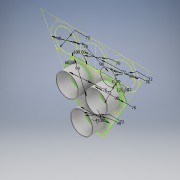
# Autodesk Inventor part: base
Saved by Autodesk Inventor 2019 (Build 230136000, 136)
## iProperties
Created: 2020-09-26
Part Number: base
Material: Generic
Document SubType Name: Modeling
Designer: Obscure_Decision
Density: 1 g/cm^3
Appearance: Default
Author: Obscure_Decision
Autodesk Inventor part; units mm, degrees
ref_plane "YZ Plane" through (0, 0, 0) normal (1, 0, 0) x (0, 1, 0)
ref_plane "XZ Plane" through (0, 0, 0) normal (0, 1, 0) x (-1, 0, 0)
ref_plane "XY Plane" through (0, 0, 0) normal (0, 0, 1) x (1, 0, 0)
sketch "Sketch1" plane through (0, 0, 0) normal (0, 0, 1) x (1, 0, 0)
  circle A0 centre (0, 0) radius 49 construction
  line L0 (0, 0) -> (49, 0) construction
  circle A1 centre (49, 84.8705) radius 49 construction
  circle A2 centre (-49, 84.8705) radius 49 construction
  circle A3 centre (0, 169.741) radius 49 construction
  circle A4 centre (-98, 169.741) radius 49 construction
  circle A5 centre (98, 169.741) radius 49 construction
  circle A6 centre (-49, 84.8705) radius 36
  circle A7 centre (-98, 169.741) radius 36 construction
  circle A8 centre (0, 169.741) radius 36 construction
  circle A9 centre (98, 169.741) radius 36 construction
  circle A10 centre (49, 84.8705) radius 36
  circle A11 centre (0, 0) radius 36
  line L1 (0, 0) -> (34.6482, -34.6482) construction
  line L2 (0, 0) -> (49, 0) construction
  line L3 (-183.7192, 220.2111) -> (183.7192, 220.2111) construction
  line L4 (-52.5602, 133.741) -> (45.4398, 133.741) construction
  line L5 (-52.5602, 133.741) -> (-77.2006, 133.741) construction
  line L6 (-52.5602, 133.741) -> (28.6753, 133.741) construction
  line L7 (45.4398, 133.741) -> (133.7957, 133.741) construction
  line L8 (45.4398, 133.741) -> (77.2264, 133.741) construction
  circle A12 centre (-49, 84.8705) radius 38
  circle A13 centre (49, 84.8705) radius 38
  circle A14 centre (0, 0) radius 38
  circle A15 centre (0, 169.741) radius 38 construction
  circle A16 centre (98, 169.741) radius 38 construction
  line L9 (-140.4352, 194.241) -> (-125.4414, 220.2111) construction
  line L10 (-140.4352, 194.241) -> (-154.5803, 169.741) construction
  line L11 (140.4352, 194.241) -> (125.4414, 220.2111) construction
  line L12 (140.4352, 194.241) -> (154.5803, 169.741) construction
  line L13 (0, -49) -> (28.2902, -49) construction
  line L14 (0, -49) -> (-28.2902, -49) construction
  line L15 (0, 207.741) -> (0, -38) construction
  circle A17 centre (-98, 169.741) radius 38 construction
  line L16 (-136, 169.741) -> (136, 169.741) construction
  line L17 (-133.7957, 133.741) -> (-183.7192, 220.2111) construction
  line L18 (133.7957, 133.741) -> (183.7192, 220.2111) construction
  line L19 (-28.2902, -49) -> (-105.4982, 84.7282) construction
  line L20 (28.2902, -49) -> (105.511, 84.7505) construction
  line L21 (-93.178, 106.0673) -> (-77.2006, 133.741) construction
  line L22 (-93.178, 106.0673) -> (-61.2232, 106.0673) construction
  line L23 (-93.178, 106.0673) -> (-105.4982, 84.7282) construction
  line L24 (-77.2006, 133.741) -> (-133.7957, 133.741) construction
  line L25 (-105.4982, 84.7282) -> (-133.7957, 133.741) construction
  line L26 (89.6177, 112.2785) -> (77.2264, 133.741) construction
  line L27 (89.6177, 112.2785) -> (114.4005, 112.2785) construction
  line L28 (89.6177, 112.2785) -> (105.511, 84.7505) construction
  line L29 (77.2264, 133.741) -> (133.7957, 133.741) construction
  line L30 (105.511, 84.7505) -> (133.7957, 133.741) construction
  line L31 (77.2264, 133.741) -> (-77.2006, 133.741) construction
  line L32 (77.2264, 133.741) -> (-77.2006, 133.741)
  line L33 (-105.4982, 84.7282) -> (-77.2006, 133.741)
  line L34 (-105.4982, 84.7282) -> (-28.2902, -49)
  line L35 (28.2902, -49) -> (-28.2902, -49)
  line L36 (28.2902, -49) -> (105.511, 84.7505)
  line L37 (77.2264, 133.741) -> (105.511, 84.7505)
  dimension "d6" = 98
  dimension "d7" = 98
  dimension "d19" = 76
  dimension "d20" = 76
  dimension "d21" = 76
  dimension "d22" = 76
  dimension "d0" = 98
  dimension "d3" = 98
  dimension "d4" = 98
  dimension "d5" = 98
  dimension "d8" = 72
  dimension "d9" = 72
  dimension "d10" = 72
  dimension "d11" = 72
  dimension "d12" = 72
  dimension "d13" = 72
  dimension "d14" = 45
  dimension "d15" = 180
  dimension "d16" = 0
  dimension "d17" = 76
  dimension "d18" = 76
  dimension "d23" = 60
  dimension "d24" = 120
  constraints: 76 end point, 13 coincident, 12 centre point, 7 collinear, 7 point on line, 6 point on circle, 2 horizontal alignment, 2 vertical alignment, 14 other
  measures "d0" diameter of A0
  measures "d3" diameter of A1
  measures "d4" diameter of A2
  measures "d5" diameter of A3
  measures "d8" diameter of A6
  measures "d9" diameter of A7
  measures "d10" diameter of A8
  measures "d11" diameter of A9
  measures "d12" diameter of A10
  measures "d13" diameter of A11
  measures "d14" angle of L1 L2
  measures "d15" angle of L5 L6
  measures "d16" distance between parallel lines of L7 L8
  measures "d17" diameter of A12
  measures "d18" diameter of A13
  measures "d23" angle of L22 L21
  measures "d24" angle of L27 L26
extrude "Extrusion1" add sketch "Sketch1" along normal blind 45 contours A12 | A13 | A14
extrude "Extrusion2" add sketch "Sketch1" against normal blind 3 contours A6 | A10 | A11 | A12 | A13 | A14 | L37 L36 L35 L34 L33 L32
sketch "Sketch2" plane through (-49, 84.8705, 0) normal (0, 0, 1) x (1, 0, 0)
  line L0 (-3, -5.5) -> (3, -5.5)
  line L1 (3, -5.5) -> (3, 5.5)
  line L2 (3, 5.5) -> (-3, 5.5)
  line L3 (-3, 5.5) -> (-3, -5.5)
  line L4 (-3, -5.5) -> (3, 5.5) construction
  line L5 (3, -5.5) -> (-3, 5.5) construction
  line L6 (94.9892, -5.5) -> (100.9892, -5.5)
  line L7 (100.9892, -5.5) -> (100.9892, 5.5)
  line L8 (100.9892, 5.5) -> (94.9892, 5.5)
  line L9 (94.9892, 5.5) -> (94.9892, -5.5)
  line L10 (94.9892, -5.5) -> (100.9892, 5.5) construction
  line L11 (100.9892, -5.5) -> (94.9892, 5.5) construction
  line L12 (46, -90.3705) -> (52, -90.3705)
  line L13 (52, -90.3705) -> (52, -79.3705)
  line L14 (52, -79.3705) -> (46, -79.3705)
  line L15 (46, -79.3705) -> (46, -90.3705)
  line L16 (46, -90.3705) -> (52, -79.3705) construction
  line L17 (52, -90.3705) -> (46, -79.3705) construction
  point P0 (49, -84.8705)
  point P1 (0, 0)
  point P2 (97.9892, 0)
  dimension "d29" = 6
  dimension "d30" = 11
  dimension "d31" = 6
  dimension "d32" = 11
  dimension "d33" = 6
  dimension "d34" = 11
  constraints: 36 end point, 6 midpoint, 6 parallel, 3 horizontal, 3 perpendicular
  measures "d29" distance of L2.end L1.end
  measures "d30" distance of L1.end L0.end
  measures "d31" distance of L8.end L7.end
  measures "d32" distance of L7.end L6.end
  measures "d33" distance of L14.end L13.end
  measures "d34" distance of L13.end L12.end
extrude "Extrusion3" cut sketch "Sketch2" against normal blind 3
body "Solid1"
